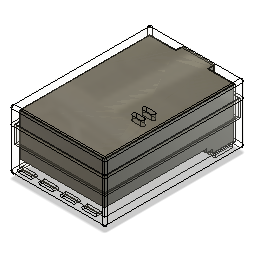
case v18 (Autodesk Fusion 360 design; units mm, degrees)
Autodesk Fusion 360 part; units mm, degrees
note: some values were not read from the file. Chosen so that the rebuilt part matches the saved one: which bodies a step acts on; which face or edge a step refers to.
sketch "Sketch1" plane through (0, 0, 0) normal (0, 1, 0) x (1, 0, 0)
  line L0 (0, 0) -> (20.1, 0)
  line L1 (20.1, 0) -> (20.1, -33.1)
  line L2 (20.1, -33.1) -> (0, -33.1)
  line L3 (0, -33.1) -> (0, 0)
  dimension "d1" = 20.1
  dimension "d2" = 33.1
  measures "d1" distance of L0.start L0.end
  measures "d2" distance of L0.start L2.end
extrude "Extrude1" add sketch "Sketch1" along normal blind 7.65 makes body 1
sketch "Sketch2" plane through (0, 7.65, 0) normal (0, 1, 0) x (-1, 0, 0)
  line L0 (0, 33.1) -> (-20.1, 33.1)
  line L1 (-20.1, 33.1) -> (-20.1, 0)
  line L2 (-20.1, 0) -> (0, 0)
  line L3 (0, 0) -> (0, 33.1)
  line L4 (-6.275, 0) -> (-13.825, 0)
  line L5 (-13.825, 0) -> (-13.825, 3.74)
  line L6 (-13.825, 3.74) -> (-6.275, 3.74)
  line L7 (-6.275, 3.74) -> (-6.275, 0)
  line L8 (-6.275, 0) -> (-13.8318, 0)
  line L9 (-6.275, 0) -> (-13.825, 0)
  line L10 (-13.825, 0) -> (-13.825, -1.76)
  line L11 (-13.825, -1.76) -> (-6.275, -1.76)
  line L12 (-6.275, -1.76) -> (-6.275, 0)
  dimension "d6" = 3.74
  dimension "d7" = 6.275
  dimension "d8" = 6.08
  dimension "d10" = 1.76
  measures "d6" distance of L4.start L6.end
  measures "d7" distance of L3 L7
  measures "d10" distance of L4.start L11.end
extrude "Extrude2" add sketch "Sketch2" against normal blind 2.75 contours L2 L4 L8 L9 L10 L11 L12 | L2 L4 L5 L6 L7 L8 L9 bodies 1
sketch "Sketch3" plane through (0, 0, 0) normal (0, -1, 0) x (1, 0, 0)
  line L0 (20.1, 33.1) -> (0, 33.1)
  line L1 (0, 33.1) -> (0, 0)
  line L2 (0, 0) -> (20.1, 0)
  line L3 (20.1, 0) -> (20.1, 33.1)
  line L4 (0, 33.1) -> (20.1, 33.1)
  line L5 (20.1, 33.1) -> (20.1, 0)
  line L6 (20.1, 0) -> (0, 0)
  line L7 (0, 0) -> (0, 33.1)
  line L8 (0, 0) -> (20.1, 0)
  line L9 (20.1, 0) -> (20.1, 6.5)
  line L10 (20.1, 6.5) -> (0, 6.5)
  line L11 (0, 6.5) -> (0, 0)
  dimension "d13" = 6.5
  measures "d13" distance of L1.end L10.end
extrude "Extrude3" add sketch "Sketch3" along normal blind 2.65 contours L0 L1 L3 L4 L5 L7 L10 bodies 1
extrude "Extrude4" add 1 faces at (6.7, 0, 2.1667) along direction (0, -1, 0) blind 4.25 on bodies 1 bodies 1
sketch "Sketch4" plane through (0, -4.25, 0) normal (0, -1, 0) x (1, 0, 0)
  line L0 (20.1, 6.5) -> (0, 6.5)
  line L1 (0, 6.5) -> (0, 0)
  line L2 (0, 0) -> (20.1, 0)
  line L3 (20.1, 0) -> (20.1, 6.5)
  line L4 (2.8, 4.3) -> (5.8, 4.3)
  line L5 (5.8, 4.3) -> (5.8, 2.75)
  line L6 (5.8, 2.75) -> (2.8, 2.75)
  line L7 (2.8, 2.75) -> (2.8, 4.3)
  line L8 (10.14, 4.3) -> (13.14, 4.3)
  line L9 (13.14, 4.3) -> (13.14, 2.75)
  line L10 (13.14, 2.75) -> (10.14, 2.75)
  line L11 (10.14, 2.75) -> (10.14, 4.3)
  line L12 (20.1, 0) -> (15.1, 0)
  line L13 (15.1, 0) -> (15.1, 5)
  line L14 (15.1, 5) -> (20.1, 5)
  line L15 (20.1, 5) -> (20.1, 0)
  dimension "d18" = 3
  dimension "d19" = 1.55
  dimension "d20" = 3
  dimension "d21" = 1.55
  dimension "d22" = 2.75
  dimension "d23" = 2.75
  dimension "d24" = 2.8
  dimension "d25" = 4.34
  dimension "d26" = 5
  dimension "d27" = 5
  measures "d18" distance of L4.start L4.end
  measures "d19" distance of L4.start L6.end
  measures "d20" distance of L8.start L8.end
  measures "d21" distance of L8.start L10.end
  measures "d22" distance of L2 L6
  measures "d23" distance of L2 L10
  measures "d24" distance of L1 L7
  measures "d25" distance of L5 L11
  measures "d26" distance of L2.end L12.end
  measures "d27" distance of L2.end L14.end
extrude "Extrude5" cut sketch "Sketch4" against normal blind 0.8 contours L0 L1 L2 L3 L13 L14 bodies 1
extrude "Extrude6" add 1 faces at (0, 4.2167, 13.2) along direction (-1, 0, 0) blind 0.1 on bodies 1 bodies 1
extrude "Extrude7" add 1 faces at (20.1, 4.2167, 13.2) along direction (1, 0, 0) blind 0.1 on bodies 1 bodies 1
extrude "Extrude8" cut 1 faces at (13.4333, 4.2167, 33.1) along direction (0, 0, -1) blind 2 on bodies 1 bodies 1
sketch "Sketch5" plane through (0, 7.65, 0) normal (0, 1, 0) x (-1, 0, 0)
  line L0 (0.1, 31.1) -> (-20.2, 31.1)
  line L1 (-20.2, 31.1) -> (-20.2, 0)
  line L2 (-20.2, 0) -> (-13.825, 0)
  line L3 (-13.825, 0) -> (-13.825, -1.76)
  line L4 (-13.825, -1.76) -> (-6.275, -1.76)
  line L5 (-6.275, -1.76) -> (-6.275, 0)
  line L6 (-6.275, 0) -> (0.1, 0)
  line L7 (0.1, 0) -> (0.1, 31.1)
  line L8 (0, 0) -> (-20.2, 0)
  line L9 (-20.2, 0) -> (-20.2, 31.1)
  line L10 (-20.2, 31.1) -> (0, 31.1)
  line L11 (0, 31.1) -> (0, 0)
  line L12 (-20.4, 31.3) -> (0.2, 31.3)
  line L13 (0.2, 31.3) -> (0.2, -0.2)
  line L14 (0.2, -0.2) -> (-20.4, -0.2)
  line L15 (-20.4, -0.2) -> (-20.4, 31.3)
  line L16 (1.4, 32.5) -> (1.4, -1.4)
  line L17 (1.4, -1.4) -> (-21.6, -1.4)
  line L18 (-21.6, -1.4) -> (-21.6, 32.5)
  line L19 (-21.6, 32.5) -> (1.4, 32.5)
  line L20 (-6.275, -0.2) -> (-6.075, -0.2)
  line L21 (-6.075, -0.2) -> (-6.075, -1.4)
  line L22 (-6.075, -1.4) -> (-6.275, -1.4)
  line L23 (-6.275, -1.4) -> (-6.275, -0.2)
  line L24 (-13.825, -0.2) -> (-14.025, -0.2)
  line L25 (-14.025, -0.2) -> (-14.025, -1.4)
  line L26 (-14.025, -1.4) -> (-13.825, -1.4)
  line L27 (-13.825, -1.4) -> (-13.825, -0.2)
  dimension "d36" = 0.2
  dimension "d37" = 1.4
  dimension "d38" = 1.2
  dimension "d43" = 0.2
  dimension "d44" = 0.2
  measures "d38" distance of L15 L18
  measures "d43" distance of L20.start L20.end
  measures "d44" distance of L24.start L24.end
extrude "Extrude9" add sketch "Sketch5" along normal blind 1.2 separate body contours L0 L1 L2 L3 L5 L6 L7 L8 L9 L10 L12 L13 L14 L15 L20 L24 | L0 L1 L2 L6 L8 L9 L10 L11 | L3 L5 L8 L14 | L5 L14 L17 L20 L21 L22 L23 | L3 L5 L14 L17 L23 L27 | L3 L14 L17 L24 L25 L26 L27 | L12 L13 L14 L15 L16 L17 L18 L19 L21 L25 makes body 2
extrude "Extrude10" add sketch "Sketch5" against normal blind 12.1 contours L12 L13 L14 L15 L16 L17 L18 L19 L21 L25 bodies 2
sketch "Sketch7" plane through (0, -4.45, 0) normal (0, -1, 0) x (1, 0, 0)
  line L0 (20.4, 31.3) -> (20.4, -0.2)
  line L1 (20.4, -0.2) -> (14.025, -0.2)
  line L2 (14.025, -0.2) -> (14.025, -1.4)
  line L3 (14.025, -1.4) -> (21.6, -1.4)
  line L4 (21.6, -1.4) -> (21.6, 32.5)
  line L5 (21.6, 32.5) -> (-1.4, 32.5)
  line L6 (-1.4, 32.5) -> (-1.4, -1.4)
  line L7 (-1.4, -1.4) -> (6.075, -1.4)
  line L8 (6.075, -1.4) -> (6.075, -0.2)
  line L9 (6.075, -0.2) -> (-0.2, -0.2)
  line L10 (-0.2, -0.2) -> (-0.2, 31.3)
  line L11 (-0.2, 31.3) -> (20.4, 31.3)
  line L12 (-1.4, 32.5) -> (21.6, 32.5)
  line L13 (21.6, 32.5) -> (21.6, -1.4)
  line L14 (21.6, -1.4) -> (-1.4, -1.4)
  line L15 (-1.4, -1.4) -> (-1.4, 32.5)
extrude "Extrude11" add sketch "Sketch7" along normal blind 1.2 bodies 2
sketch "Sketch8" plane through (0, -4.45, 0) normal (0, 1, 0) x (-1, 0, 0)
  line L0 (-6.075, -1.4) -> (-6.075, -0.2)
  line L1 (-6.075, -0.2) -> (0.2, -0.2)
  line L2 (0.2, -0.2) -> (0.2, 31.3)
  line L3 (0.2, 31.3) -> (-20.4, 31.3)
  line L4 (-20.4, 31.3) -> (-20.4, -0.2)
  line L5 (-20.4, -0.2) -> (-14.025, -0.2)
  line L6 (-14.025, -0.2) -> (-14.025, -1.4)
  line L7 (-14.025, -1.4) -> (-6.075, -1.4)
  line L8 (-6.075, -1.4) -> (-14.025, -1.4)
  line L9 (-14.025, -1.4) -> (-14.025, -0.2)
  line L10 (-14.025, -0.2) -> (-6.075, -0.2)
  line L11 (-6.075, -0.2) -> (-6.075, -1.4)
extrude "Extrude12" add sketch "Sketch8" along normal blind 9.15 contours L0 L6 L7 L8 L9 L10 L11 bodies 2
fillet "Fillet1" radius 0.6 4 edges at (-1.4, 1.6, 32.5) (21.6, 1.6, 32.5) (21.6, 1.6, -1.4) (-1.4, 1.6, -1.4) on bodies 2
fillet "Fillet2" radius 0.6 16 edges at (10.1, 8.85, -1.4) (21.4243, 8.85, -1.2243) (21.6, 8.85, 15.55) (21.4243, 8.85, 32.3243) (10.1, 8.85, 32.5) (-1.2243, 8.85, 32.3243) (-1.4, 8.85, 15.55) (-1.2243, 8.85, -1.2243) (-1.2243, -5.65, -1.2243) (10.1, -5.65, -1.4) (21.4243, -5.65, -1.2243) (21.6, -5.65, 15.55) (21.4243, -5.65, 32.3243) (10.1, -5.65, 32.5) (-1.2243, -5.65, 32.3243) (-1.4, -5.65, 15.55) on bodies 2
copy_body "Body->Comp1" bodies 1 removing the originals makes body 3 in component "Electronics"
copy_body "Body->Comp2" bodies 2 removing the originals makes body 4 in component "Case"
sketch "Sketch2 (2)" plane through (0, -5.65, 0) normal (0, -1, 0) x (1, 0, 0) in component "Case"
  line L0 (-0.8, 31.9) -> (-0.8, -0.8)
  line L1 (-0.8, -0.8) -> (21, -0.8)
  line L2 (21, -0.8) -> (21, 31.9)
  line L3 (21, 31.9) -> (-0.8, 31.9)
  line L4 (21, -0.8) -> (15, -0.8)
  line L5 (15, -0.8) -> (15, 5.2)
  line L6 (15, 5.2) -> (21, 5.2)
  line L7 (21, 5.2) -> (21, -0.8)
  line L8 (15, 0.2) -> (21, 0.2)
  line L9 (21, 4.2) -> (15, 4.2)
  line L10 (16.2, 4.2) -> (16.2, 0.2)
  line L11 (17.4, 0.2) -> (17.4, 4.2)
  line L12 (18.6, 4.2) -> (18.6, 0.2)
  line L13 (19.8, 4.2) -> (19.8, 0.2)
  line L14 (15.9, 4.2) -> (15.9, 0.2)
  arc A0 (15.9, 0.2) -> (16.5, 0.2) centre (16.2, 0.2) ccw
  line L15 (16.5, 0.2) -> (16.5, 4.2)
  arc A1 (16.5, 4.2) -> (15.9, 4.2) centre (16.2, 4.2) ccw
  line L16 (16.2, 4.2) -> (16.2, 0.2) construction
  line L17 (17.7, 0.2) -> (17.7, 4.2)
  arc A2 (17.7, 4.2) -> (17.1, 4.2) centre (17.4, 4.2) ccw
  line L18 (17.1, 4.2) -> (17.1, 0.2)
  arc A3 (17.1, 0.2) -> (17.7, 0.2) centre (17.4, 0.2) ccw
  line L19 (17.4, 0.2) -> (17.4, 4.2) construction
  line L20 (18.3, 4.2) -> (18.3, 0.2)
  arc A4 (18.3, 0.2) -> (18.9, 0.2) centre (18.6, 0.2) ccw
  line L21 (18.9, 0.2) -> (18.9, 4.2)
  arc A5 (18.9, 4.2) -> (18.3, 4.2) centre (18.6, 4.2) ccw
  line L22 (18.6, 4.2) -> (18.6, 0.2) construction
  line L23 (19.5, 4.2) -> (19.5, 0.2)
  arc A6 (19.5, 0.2) -> (20.1, 0.2) centre (19.8, 0.2) ccw
  line L24 (20.1, 0.2) -> (20.1, 4.2)
  arc A7 (20.1, 4.2) -> (19.5, 4.2) centre (19.8, 4.2) ccw
  line L25 (19.8, 4.2) -> (19.8, 0.2) construction
  dimension "d64" = 6
  dimension "d65" = 6
  dimension "d66" = 1
  dimension "d67" = 1
  dimension "d68" = 1.2
  dimension "d69" = 1.2
  dimension "d70" = 1.2
  dimension "d71" = 1.2
  dimension "d72" = 1.2
  dimension "d74" = 0.6
  dimension "d75" = 0.6
  dimension "d76" = 0.6
  dimension "d77" = 0.6
  measures "d64" distance of L1.end L4.end
  measures "d65" distance of L1.end L6.end
  measures "d66" distance of L6 L9
  measures "d67" distance of L4 L8
  measures "d68" distance of L5 L10
  measures "d69" distance of L10 L11
  measures "d70" distance of L7 L13
  measures "d71" distance of L12 L13
  measures "d72" distance of L11 L12
  measures "d74" diameter of A0
  measures "d75" diameter of A2
  measures "d76" diameter of A4
  measures "d77" diameter of A6
extrude "Extrude1'" cut sketch "Sketch2 (2)" against normal blind 1.2 contours L8 L9 L10 L14 | L8 A0 | L8 L9 L13 L24 | L9 A7 | L8 A6 | L9 A1 | L8 L9 L10 L15 | L8 L9 L13 L23 | L8 L9 L11 L18 | L8 A3 | L8 L9 L12 L21 | L9 A5 | L8 A4 | L9 A2 | L8 L9 L11 L17 | L8 L9 L12 L20 bodies 4 in component "Case"
extrude "Extrude2'" cut sketch "Sketch4" along normal blind 8 contours L4 L5 L6 L7 | L8 L9 L10 L11 bodies 4 in component "Case"
sketch "Sketch9" plane through (0, -4.45, 0) normal (0, 1, 0) x (-1, 0, 0)
  line L0 (-2.8, 4.3) -> (-2.8, 2.75)
  line L1 (-2.8, 2.75) -> (-5.8, 2.75)
  line L2 (-5.8, 2.75) -> (-5.8, 4.3)
  line L3 (-5.8, 4.3) -> (-2.8, 4.3)
  line L4 (-10.14, 4.3) -> (-10.14, 2.75)
  line L5 (-10.14, 2.75) -> (-13.14, 2.75)
  line L6 (-13.14, 2.75) -> (-13.14, 4.3)
  line L7 (-13.14, 4.3) -> (-10.14, 4.3)
  line L8 (-17.7, 0.2) -> (-17.7, 4.2)
  arc A0 (-17.1, 4.2) -> (-17.7, 4.2) centre (-17.4, 4.2) ccw
  line L9 (-17.1, 4.2) -> (-17.1, 0.2)
  arc A1 (-17.7, 0.2) -> (-17.1, 0.2) centre (-17.4, 0.2) ccw
  line L10 (-18.3, 4.2) -> (-18.3, 0.2)
  arc A2 (-18.9, 0.2) -> (-18.3, 0.2) centre (-18.6, 0.2) ccw
  line L11 (-18.9, 0.2) -> (-18.9, 4.2)
  arc A3 (-18.3, 4.2) -> (-18.9, 4.2) centre (-18.6, 4.2) ccw
  line L12 (-15.9, 4.2) -> (-15.9, 0.2)
  arc A4 (-16.5, 0.2) -> (-15.9, 0.2) centre (-16.2, 0.2) ccw
  line L13 (-16.5, 0.2) -> (-16.5, 4.2)
  arc A5 (-15.9, 4.2) -> (-16.5, 4.2) centre (-16.2, 4.2) ccw
  line L14 (-19.5, 4.2) -> (-19.5, 0.2)
  arc A6 (-20.1, 0.2) -> (-19.5, 0.2) centre (-19.8, 0.2) ccw
  line L15 (-20.1, 0.2) -> (-20.1, 4.2)
  arc A7 (-19.5, 4.2) -> (-20.1, 4.2) centre (-19.8, 4.2) ccw
  line L16 (-20.4, -0.2) -> (0.2, -0.2)
  line L17 (0.2, -0.2) -> (0.2, 31.3)
  line L18 (0.2, 31.3) -> (-20.4, 31.3)
  line L19 (-20.4, 31.3) -> (-20.4, -0.2)
  line L20 (-1.8, 5.3) -> (-1.8, 1.75)
  line L21 (-1.8, 1.75) -> (-6.8, 1.75)
  line L22 (-6.8, 1.75) -> (-6.8, 5.3)
  line L23 (-6.8, 5.3) -> (-1.8, 5.3)
  line L24 (-14.14, 5.3) -> (-9.14, 5.3)
  line L25 (-9.14, 5.3) -> (-9.14, 1.75)
  line L26 (-9.14, 1.75) -> (-14.14, 1.75)
  line L27 (-14.14, 1.75) -> (-14.14, 5.3)
  dimension "d84" = 1
  dimension "d85" = 1
extrude "Extrude3'" cut sketch "Sketch9" against normal blind 0.7 contours L20 L21 L22 L23 | L24 L25 L26 L27 bodies 4 in component "Case"
sketch "Sketch10" plane through (0, -4.45, 0) normal (0, 1, 0) x (-1, 0, 0)
  line L0 (-1.8, 1.75) -> (-6.8, 1.75)
  line L1 (-6.8, 1.75) -> (-6.8, 5.3)
  line L2 (-6.8, 5.3) -> (-1.8, 5.3)
  line L3 (-1.8, 5.3) -> (-1.8, 1.75)
  line L4 (-9.14, 5.3) -> (-9.14, 1.75)
  line L5 (-9.14, 1.75) -> (-14.14, 1.75)
  line L6 (-14.14, 1.75) -> (-14.14, 5.3)
  line L7 (-14.14, 5.3) -> (-9.14, 5.3)
  line L8 (-17.7, 0.2) -> (-17.7, 4.2)
  arc A0 (-17.1, 4.2) -> (-17.7, 4.2) centre (-17.4, 4.2) ccw
  line L9 (-17.1, 4.2) -> (-17.1, 0.2)
  arc A1 (-17.7, 0.2) -> (-17.1, 0.2) centre (-17.4, 0.2) ccw
  line L10 (-18.3, 4.2) -> (-18.3, 0.2)
  arc A2 (-18.9, 0.2) -> (-18.3, 0.2) centre (-18.6, 0.2) ccw
  line L11 (-18.9, 0.2) -> (-18.9, 4.2)
  arc A3 (-18.3, 4.2) -> (-18.9, 4.2) centre (-18.6, 4.2) ccw
  line L12 (-15.9, 4.2) -> (-15.9, 0.2)
  arc A4 (-16.5, 0.2) -> (-15.9, 0.2) centre (-16.2, 0.2) ccw
  line L13 (-16.5, 0.2) -> (-16.5, 4.2)
  arc A5 (-15.9, 4.2) -> (-16.5, 4.2) centre (-16.2, 4.2) ccw
  line L14 (-19.5, 4.2) -> (-19.5, 0.2)
  arc A6 (-20.1, 0.2) -> (-19.5, 0.2) centre (-19.8, 0.2) ccw
  line L15 (-20.1, 0.2) -> (-20.1, 4.2)
  arc A7 (-19.5, 4.2) -> (-20.1, 4.2) centre (-19.8, 4.2) ccw
  line L16 (-20.4, -0.2) -> (0.2, -0.2)
  line L17 (0.2, -0.2) -> (0.2, 31.3)
  line L18 (0.2, 31.3) -> (-20.4, 31.3)
  line L19 (-20.4, 31.3) -> (-20.4, -0.2)
  line L20 (-2, 5.1) -> (-2, 1.95)
  line L21 (-2, 1.95) -> (-6.6, 1.95)
  line L22 (-6.6, 1.95) -> (-6.6, 5.1)
  line L23 (-6.6, 5.1) -> (-2, 5.1)
  line L24 (-13.94, 1.95) -> (-13.94, 5.1)
  line L25 (-13.94, 5.1) -> (-9.34, 5.1)
  line L26 (-9.34, 5.1) -> (-9.34, 1.95)
  line L27 (-9.34, 1.95) -> (-13.94, 1.95)
  line L28 (-2.8, 4.3) -> (-5.8, 4.3)
  line L29 (-5.8, 4.3) -> (-5.8, 2.75)
  line L30 (-5.8, 2.75) -> (-2.8, 2.75)
  line L31 (-2.8, 2.75) -> (-2.8, 4.3)
  line L32 (-10.14, 4.3) -> (-13.14, 4.3)
  line L33 (-13.14, 4.3) -> (-13.14, 2.75)
  line L34 (-13.14, 2.75) -> (-10.14, 2.75)
  line L35 (-10.14, 2.75) -> (-10.14, 4.3)
  line L36 (-5.6, 2.95) -> (-3, 2.95)
  line L37 (-3, 2.95) -> (-3, 4.1)
  line L38 (-3, 4.1) -> (-5.6, 4.1)
  line L39 (-5.6, 4.1) -> (-5.6, 2.95)
  line L40 (-10.34, 4.1) -> (-12.94, 4.1)
  line L41 (-12.94, 4.1) -> (-12.94, 2.95)
  line L42 (-12.94, 2.95) -> (-10.34, 2.95)
  line L43 (-10.34, 2.95) -> (-10.34, 4.1)
  point P0 (-2.8, 4.3)
  point P1 (-5.8, 2.75)
  point P2 (-10.14, 4.3)
  point P3 (-13.14, 2.75)
  dimension "d88" = 0.2
  dimension "d89" = 0.2
  dimension "d94" = 0.2
  dimension "d95" = 0.2
extrude "Extrude13" add sketch "Sketch10" against normal blind 0.5 separate body contours L20 L21 L22 L23 | L24 L25 L26 L27 makes body 5 at (4.8, -4.45, 2.2167) makes body 6 at (12.14, -4.45, 2.2167)
extrude "Extrude15" add sketch "Sketch10" against normal blind 0.5 contours L28 L29 L30 L31 | L32 L33 L34 L35 | L36 L37 L38 L39 | L40 L41 L42 L43 bodies 5 6
extrude "Extrude16" add sketch "Sketch10" against normal blind 1.6 contours L36 L37 L38 L39 | L40 L41 L42 L43 bodies 5 6
extrude "Extrude17" add 2 faces at (4.7333, -6.05, 3.7167) (11.2067, -6.05, 3.7167) along direction (0, -1, 0) blind 0.4 on bodies 5 6 bodies 5 6
ref_plane "WorkPlane1" through (10.05, 4.7, -0.8) normal (0, 1, 0) x (0, 0, 1)
copy_body "Body->Comp3" bodies 6 removing the originals makes body 7 in component "button1"
copy_body "Body->Comp4" bodies 5 removing the originals makes body 8 in component "button2"
split "Split1" by plane through (10.05, 4.7, -0.8) normal (0, 1, 0) bodies 4 makes body 9 at (14, 8.85, 20.7333) in component "Case"
sketch "seam Sketch" plane through (0, 4.7, 0) normal (0, 1, 0) x (-1, 0, 0) in component "Case"
  line L0 (0.2, -0.2) -> (-20.4, -0.2)
  line L1 (-20.4, -0.2) -> (-20.4, 31.3)
  line L2 (-20.4, 31.3) -> (0.2, 31.3)
  line L3 (0.2, 31.3) -> (0.2, -0.2)
  line L4 (-21, -1.4) -> (0.8, -1.4)
  arc A0 (0.8, -1.4) -> (1.4, -0.8) centre (0.8, -0.8) ccw
  line L5 (1.4, -0.8) -> (1.4, 31.9)
  arc A1 (1.4, 31.9) -> (0.8, 32.5) centre (0.8, 31.9) ccw
  line L6 (0.8, 32.5) -> (-21, 32.5)
  arc A2 (-21, 32.5) -> (-21.6, 31.9) centre (-21, 31.9) ccw
  line L7 (-21.6, 31.9) -> (-21.6, -0.8)
  arc A3 (-21.6, -0.8) -> (-21, -1.4) centre (-21, -0.8) ccw
  line L8 (0.2, -0.2) -> (-20.4, -0.2)
  line L9 (-20.4, -0.2) -> (-20.4, 31.3)
  line L10 (-20.4, 31.3) -> (0.2, 31.3)
  line L11 (0.2, 31.3) -> (0.2, -0.2)
  line L12 (0.8, -0.8) -> (0.8, 31.9)
  line L13 (-20.8, 31.7) -> (0.6, 31.7)
  line L14 (0.6, 31.7) -> (0.6, -0.6)
  line L15 (0.6, -0.6) -> (-20.8, -0.6)
  line L16 (-20.8, -0.6) -> (-20.8, 31.7)
  line L17 (0.8, 31.9) -> (-21, 31.9)
  line L18 (-21, 31.9) -> (-21, -0.8)
  line L19 (-21, -0.8) -> (0.8, -0.8)
  line L20 (0.8, -0.8) -> (0.8, 31.9)
  dimension "d112" = 0.6
  dimension "d113" = 0.6
  dimension "d114" = 0.4
  measures "d112" distance of L5 L12
  measures "d113" distance of L11 L12
extrude "Extrude7'" add sketch "seam Sketch" against normal blind 4 contours L13 L14 L15 L16 bodies 9 in component "Case"
extrude "Extrude8'" cut sketch "seam Sketch" against normal blind 4.2 contours L13 L14 L15 L16 bodies 4 in component "Case"
extrude "Extrude9'" cut sketch "seam Sketch" against normal blind 4.2 contours L12 L17 L18 L19 L20 | L13 L14 L15 L16 bodies 4 in component "Case"
extrude "Extrude6'" add 1 faces at (0, 8.45, 20.7333) along direction (-1, 0, 0) blind 0.1 on bodies 9 bodies 9 in component "Case"
extrude "Extrude10'" cut 1 faces at (8.725, 4.7, -0.4667) along direction (0, -1, 0) blind 4 on bodies 9 bodies 9 in component "Case"
sketch "Sketch5 (2)" plane through (0, 4.7, 0) normal (0, -1, 0) x (1, 0, 0) in component "Case"
  line L0 (20.8, -0.6) -> (14.025, -0.6)
  line L1 (14.025, -0.6) -> (14.025, -1.4)
  line L2 (14.025, -1.4) -> (21, -1.4)
  arc A0 (21, -1.4) -> (21.6, -0.8) centre (21, -0.8) ccw
  line L3 (21.6, -0.8) -> (21.6, 31.9)
  arc A1 (21.6, 31.9) -> (21, 32.5) centre (21, 31.9) ccw
  line L4 (21, 32.5) -> (-0.8, 32.5)
  arc A2 (-0.8, 32.5) -> (-1.4, 31.9) centre (-0.8, 31.9) ccw
  line L5 (-1.4, 31.9) -> (-1.4, -0.8)
  arc A3 (-1.4, -0.8) -> (-0.8, -1.4) centre (-0.8, -0.8) ccw
  line L6 (-0.8, -1.4) -> (6.075, -1.4)
  line L7 (6.075, -1.4) -> (6.075, -0.6)
  line L8 (6.075, -0.6) -> (-0.6, -0.6)
  line L9 (-0.6, -0.6) -> (-0.6, 31.7)
  line L10 (-0.6, 31.7) -> (20.8, 31.7)
  line L11 (20.8, 31.7) -> (20.8, -0.6)
  line L12 (6.075, -1.4) -> (14.025, -1.4)
  line L13 (14.025, -1.4) -> (14.025, -0.6)
  line L14 (14.025, -0.6) -> (6.075, -0.6)
  line L15 (6.075, -0.6) -> (6.075, -1.4)
  line L16 (6.275, -0.6) -> (6.275, -1.4)
  line L17 (13.825, -0.6) -> (13.825, -1.4)
  dimension "d123" = 0.2
  dimension "d124" = 0.2
  measures "d123" distance of L15 L16
  measures "d124" distance of L13 L17
extrude "Extrude11'" add sketch "Sketch5 (2)" along normal blind 4.2 contours L12 L14 L16 L17 bodies 4 in component "Case"
extrude "Extrude12'" add 1 faces at (11.3083, 3.3, -0.6) along direction (0, 0, 1) blind 0.4 on bodies 4 bodies 4 in component "Case"
sketch "Sketch11" plane through (0, 0, 32.5) normal (0, 0, 1) x (1, 0, 0)
  line L0 (21, 4.7) -> (-0.8, 4.7)
  line L1 (-0.8, 4.7) -> (-0.8, -5.05)
  line L2 (-0.8, -5.05) -> (21, -5.05)
  line L3 (21, -5.05) -> (21, 4.7)
  line L4 (-0.2, -4.45) -> (20.4, -4.45)
  line L5 (-0.2, 0.5) -> (-0.2, -4.45)
  line L6 (20.4, 0.5) -> (20.4, -4.45)
  line L7 (0.8, -3.95) -> (19.4, -3.95)
  line L8 (0.8, -4.25) -> (3.8, -4.25)
  arc A0 (3.8, -4.25) -> (3.8, -3.65) centre (3.8, -3.95) ccw
  line L9 (3.8, -3.65) -> (0.8, -3.65)
  arc A1 (0.8, -3.65) -> (0.8, -4.25) centre (0.8, -3.95) ccw
  line L10 (0.8, -3.95) -> (3.8, -3.95) construction
  line L11 (6, -4.25) -> (9, -4.25)
  arc A2 (9, -4.25) -> (9, -3.65) centre (9, -3.95) ccw
  line L12 (9, -3.65) -> (6, -3.65)
  arc A3 (6, -3.65) -> (6, -4.25) centre (6, -3.95) ccw
  line L13 (6, -3.95) -> (9, -3.95) construction
  line L14 (11.2, -4.25) -> (14.2, -4.25)
  arc A4 (14.2, -4.25) -> (14.2, -3.65) centre (14.2, -3.95) ccw
  line L15 (14.2, -3.65) -> (11.2, -3.65)
  arc A5 (11.2, -3.65) -> (11.2, -4.25) centre (11.2, -3.95) ccw
  line L16 (11.2, -3.95) -> (14.2, -3.95) construction
  line L17 (16.4, -4.25) -> (19.4, -4.25)
  arc A6 (19.4, -4.25) -> (19.4, -3.65) centre (19.4, -3.95) ccw
  line L18 (19.4, -3.65) -> (16.4, -3.65)
  arc A7 (16.4, -3.65) -> (16.4, -4.25) centre (16.4, -3.95) ccw
  line L19 (16.4, -3.95) -> (19.4, -3.95) construction
  point P0 (0.8, -3.95)
  point P1 (19.4, -3.95)
  point P2 (3.8, -3.95)
  point P3 (6, -3.95)
  point P4 (9, -3.95)
  point P5 (11.2, -3.95)
  point P6 (14.2, -3.95)
  point P7 (16.4, -3.95)
  point P8 (10.1, -3.95)
  dimension "d130" = 1
  dimension "d132" = 1
  dimension "d133" = 1.1
  dimension "d134" = 1.1
  dimension "d135" = 18.6
  dimension "d138" = 3
  dimension "d139" = 3
  dimension "d140" = 1.1
  dimension "d141" = 1.1
  dimension "d142" = 3
  dimension "d143" = 2.2
  dimension "d144" = 2.3
  dimension "d145" = 3.3
  dimension "d146" = 0.6
  dimension "d147" = 0.6
  dimension "d148" = 0.6
  dimension "d149" = 0.6
  measures "d130" distance of P0 L5
  measures "d132" distance of P1 L6
  measures "d133" distance of L2 P0
  measures "d134" distance of L2 P1
  measures "d135" distance of P0 P1
  measures "d138" distance of P0 P2
  measures "d139" distance of P3 P4
  measures "d140" distance of P4 P8
  measures "d141" distance of P5 P8
  measures "d142" distance of P5 P6
  measures "d143" distance of P6 P7
  measures "d146" diameter of A0
  measures "d147" diameter of A2
  measures "d148" diameter of A4
  measures "d149" diameter of A6
extrude "Extrude13'" cut sketch "Sketch11" against normal blind 1.2 contours L7 A2 L12 A3 | L7 L11 A2 A3 | L7 A4 L15 A5 | L7 L14 A4 A5 | L8 A0 L9 A1 | L17 A6 L18 A7 bodies 4 in component "Case"
sketch "Sketch12" plane through (0, -5.65, 0) normal (0, -1, 0) x (1, 0, 0)
  line L0 (2.8, 2.75) -> (2.8, 4.3)
  line L1 (2.8, 4.3) -> (5.8, 4.3)
  line L2 (5.8, 4.3) -> (5.8, 2.75)
  line L3 (5.8, 2.75) -> (2.8, 2.75)
  line L4 (10.14, 2.75) -> (10.14, 4.3)
  line L5 (10.14, 4.3) -> (13.14, 4.3)
  line L6 (13.14, 4.3) -> (13.14, 2.75)
  line L7 (13.14, 2.75) -> (10.14, 2.75)
  line L8 (17.7, 4.2) -> (17.7, 0.2)
  arc A0 (17.1, 0.2) -> (17.7, 0.2) centre (17.4, 0.2) ccw
  line L9 (17.1, 0.2) -> (17.1, 4.2)
  arc A1 (17.7, 4.2) -> (17.1, 4.2) centre (17.4, 4.2) ccw
  line L10 (18.3, 0.2) -> (18.3, 4.2)
  arc A2 (18.9, 4.2) -> (18.3, 4.2) centre (18.6, 4.2) ccw
  line L11 (18.9, 4.2) -> (18.9, 0.2)
  arc A3 (18.3, 0.2) -> (18.9, 0.2) centre (18.6, 0.2) ccw
  line L12 (15.9, 0.2) -> (15.9, 4.2)
  arc A4 (16.5, 4.2) -> (15.9, 4.2) centre (16.2, 4.2) ccw
  line L13 (16.5, 4.2) -> (16.5, 0.2)
  arc A5 (15.9, 0.2) -> (16.5, 0.2) centre (16.2, 0.2) ccw
  line L14 (19.5, 0.2) -> (19.5, 4.2)
  arc A6 (20.1, 4.2) -> (19.5, 4.2) centre (19.8, 4.2) ccw
  line L15 (20.1, 4.2) -> (20.1, 0.2)
  arc A7 (19.5, 0.2) -> (20.1, 0.2) centre (19.8, 0.2) ccw
  line L16 (-0.8, -0.8) -> (21, -0.8)
  line L17 (21, -0.8) -> (21, 31.9)
  line L18 (21, 31.9) -> (-0.8, 31.9)
  line L19 (-0.8, 31.9) -> (-0.8, -0.8)
  line L20 (-0.1, 31.1) -> (20.1, 31.1)
  line L21 (20.1, 31.1) -> (20.1, 0.2)
  line L22 (20.1, 0.2) -> (-0.1, 0.2)
  line L23 (-0.1, 0.2) -> (-0.1, 31.1)
  line L24 (11.6001, 22.1) -> (11.6001, 23.1)
  arc A8 (11.6001, 23.1) -> (10.5999, 23.1) centre (11.1, 23.1) ccw
  line L25 (10.5999, 23.1) -> (10.5999, 22.1)
  arc A9 (10.5999, 22.1) -> (11.6001, 22.1) centre (11.1, 22.1) ccw
  line L26 (11.1, 22.1) -> (11.1, 23.1) construction
  point P0 (-0.1, 31.1)
  point P1 (11.1, 22.6)
  point P2 (11.1, 22.6)
  dimension "d152" = 8.5
  dimension "d153" = 11.2
  dimension "d154" = 9
  dimension "d155" = 1
  measures "d152" distance of L20 P2
  measures "d153" distance of L23 P2
  measures "d154" distance of L21 P2
  measures "d155" distance of A9.centre A8.centre
extrude "Extrude14" cut sketch "Sketch12" against normal blind 1.2 contours L24 A8 L25 A9 bodies 4 in component "Case"
sketch "Sketch13" plane through (0, 8.85, 0) normal (0, 1, 0) x (-1, 0, 0)
  line L0 (-21, 31.9) -> (-21, -0.8)
  line L1 (-21, -0.8) -> (0.8, -0.8)
  line L2 (0.8, -0.8) -> (0.8, 31.9)
  line L3 (0.8, 31.9) -> (-21, 31.9)
  line L4 (-13.825, 0) -> (-20.2, 0)
  line L5 (-20.2, 0) -> (-20.2, 31.1)
  line L6 (-15.8, 17.5) -> (-17.8, 17.5)
  arc A0 (-17.8, 17.5) -> (-17.8, 16.5) centre (-17.8, 17) ccw
  line L7 (-17.8, 16.5) -> (-15.8, 16.5)
  arc A1 (-15.8, 16.5) -> (-15.8, 17.5) centre (-15.8, 17) ccw
  line L8 (-15.8, 17) -> (-17.8, 17) construction
  line L9 (-15.8, 20) -> (-17.8, 20)
  arc A2 (-17.8, 20) -> (-17.8, 19) centre (-17.8, 19.5) ccw
  line L10 (-17.8, 19) -> (-15.8, 19)
  arc A3 (-15.8, 19) -> (-15.8, 20) centre (-15.8, 19.5) ccw
  line L11 (-15.8, 19.5) -> (-17.8, 19.5) construction
  point P0 (-16.8, 17)
  point P1 (-16.8, 19.5)
  point P2 (-16.8, 17)
  point P3 (-16.8, 19.5)
  dimension "d158" = 17
  dimension "d159" = 2.5
  dimension "d160" = 3.4
  dimension "d161" = 3.4
  dimension "d162" = 1
  measures "d158" distance of P2 L4
  measures "d159" distance of P2 P3
  measures "d160" distance of P2 L5
  measures "d161" distance of P3 L5
  measures "d162" diameter of A0
extrude "Extrude15'" cut sketch "Sketch13" against normal blind 1.2 contours L6 A0 L7 A1 | L9 A2 L10 A3 bodies 9 in component "Case"
extrude "Extrude1''" add 1 faces at (4.7333, -6.45, 3.7167) along direction (0, -1, 0) blind 0.2 on bodies 8 bodies 8 in component "button2"
extrude "Extrude1'''" add 1 faces at (11.2067, -6.45, 3.7167) along direction (0, -1, 0) blind 0.2 on bodies 7 bodies 7 in component "button1"
component "Electronics" placed x (1, 0, 0) y (0, 1, 0) z (0, 0, 1) at (0, 0, 0)
component "Case" placed x (1, 0, 0) y (0, 1, 0) z (0, 0, 1) at (0, 0, 0)
component "button1" placed x (1, 0, 0) y (0, 1, 0) z (0, 0, 1) at (0, 0, 0)
component "button2" placed x (1, 0, 0) y (0, 1, 0) z (0, 0, 1) at (0, 0, 0)
equation "slot = 0.6 mm"
equation "d74 = slot"
equation "d75 = slot"
equation "d76 = slot"
equation "d77 = slot"
equation "slot_size = 3 mm"
equation "slot_spacing = 2.2 mm"
equation "d138 = slot_size"
equation "d139 = slot_size"
equation "d140 = slot_spacing / 2"
equation "d141 = slot_spacing / 2"
equation "d142 = slot_size"
equation "d143 = slot_spacing"
equation "d146 = slot"
equation "d147 = slot"
equation "d148 = slot"
equation "d149 = slot"
named bodies: "Electronics", "Case", "Case top", "Case bottom"
